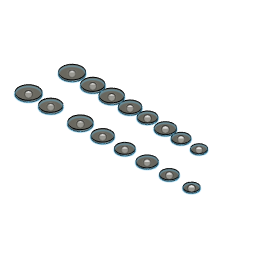
Euro As STL Cylinder v1 (Autodesk Fusion 360 design; units mm, degrees)
Autodesk Fusion 360 part; units mm, degrees
sketch "Esquisse1" plane through (0, 0, 0) normal (0, 0, 1) x (1, 0, 0)
  circle A0 centre (5.5632, 13.2312) radius 12.875
  circle A1 centre (34.0041, 12.6972) radius 11.6
  circle A2 centre (59.7259, 12.4935) radius 12.125
  circle A3 centre (85.1004, 11.9486) radius 11.125
  circle A4 centre (108.6293, 11.9434) radius 9.85
  circle A5 centre (133.4711, 11.2171) radius 10.64
  circle A6 centre (155.5746, 10.2389) radius 9.4
  circle A7 centre (180.0756, 9.9611) radius 8.125
  circle A8 centre (0, -40) radius 12.875
  circle A9 centre (30, -40) radius 11.625
  circle A10 centre (70, -40) radius 12.125
  circle A11 centre (100, -40) radius 11.125
  circle A12 centre (130, -40) radius 9.875
  circle A13 centre (160, -40) radius 10.625
  circle A14 centre (190, -40) radius 9.375
  circle A15 centre (220, -40) radius 8.125
  dimension "d1" = 25.75
  dimension "d2" = 23.2
  dimension "d3" = 24.25
  dimension "d4" = 22.25
  dimension "d5" = 19.7
  dimension "d6" = 21.28
  dimension "d7" = 18.8
  dimension "d8" = 16.25
  dimension "d25" = 25.75
  dimension "d26" = 23.25
  dimension "d27" = 24.25
  dimension "d28" = 22.25
  dimension "d29" = 19.75
  dimension "d30" = 21.25
  dimension "d31" = 18.75
  dimension "d32" = 16.25
  measures "d1" diameter of A0
  measures "d2" diameter of A1
  measures "d3" diameter of A2
  measures "d4" diameter of A3
  measures "d5" diameter of A4
  measures "d6" diameter of A5
  measures "d7" diameter of A6
  measures "d8" diameter of A7
  measures "d25" diameter of A8
  measures "d26" diameter of A9
  measures "d27" diameter of A10
  measures "d28" diameter of A11
  measures "d29" diameter of A12
  measures "d30" diameter of A13
  measures "d31" diameter of A14
  measures "d32" diameter of A15
extrude "Extrusion1" add sketch "Esquisse1" along normal blind 2.2 contours A0 makes body 1
extrude "Extrusion2" add sketch "Esquisse1" along normal blind 2.4 separate body contours A1 makes body 2
extrude "Extrusion3" add sketch "Esquisse1" along normal blind 2.33 separate body contours A2 makes body 3
extrude "Extrusion4" add sketch "Esquisse1" along normal blind 2.1 separate body contours A3 makes body 4
extrude "Extrusion5" add sketch "Esquisse1" along normal blind 1.9 separate body contours A4 makes body 5
extrude "Extrusion6" add sketch "Esquisse1" along normal blind 1.65 separate body contours A5 makes body 6
extrude "Extrusion7" add sketch "Esquisse1" along normal blind 1.65 separate body contours A6 makes body 7
extrude "Extrusion8" add sketch "Esquisse1" along normal blind 1.6 separate body contours A7 makes body 8
extrude "Extrusion9" add sketch "Esquisse1" along normal blind 1.67 separate body contours A15 makes body 9
extrude "Extrusion10" add sketch "Esquisse1" along normal blind 1.67 separate body contours A14 makes body 10
extrude "Extrusion11" add sketch "Esquisse1" along normal blind 1.67 separate body contours A13 makes body 11
extrude "Extrusion12" add sketch "Esquisse1" along normal blind 1.93 separate body contours A12 makes body 12
extrude "Extrusion13" add sketch "Esquisse1" along normal blind 2.14 separate body contours A11 makes body 13
extrude "Extrusion14" add sketch "Esquisse1" along normal blind 2.38 separate body contours A10 makes body 14
extrude "Extrusion15" add sketch "Esquisse1" along normal blind 2.33 separate body contours A9 makes body 15
extrude "Extrusion16" add sketch "Esquisse1" along normal blind 2.2 separate body contours A8 makes body 16
sketch "Esquisse2" plane through (0, 0, 0) normal (0, 0, 1) x (1, 0, 0)
named bodies: "2E", "1E", "50Cent", "20Cent", "10Cent", "5Cent", "2Cent", "1Cent", "1CentOfficial", "2CentOfficial", "5CentOfficial", "10CentOfficial", "20CentOfficial", "50CentOfficial", "1EuroOfficial", "2EuroOfficial"
